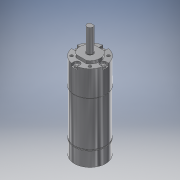
# Autodesk Inventor part: 730RPM Motor Mockup
Saved by Autodesk Inventor 2017 (Build 210142000, 142)
## iProperties
Created: 2019-01-30
Part Number: 730RPM Motor Mockup
Material: Generic
Document SubType Name: Modeling
Designer: cresswnd
Density: 1 g/cm^3
Appearance: Aluminum - Polished
Author: cresswnd
Autodesk Inventor part; units mm, degrees
ref_plane "YZ Plane" through (0, 0, 0) normal (1, 0, 0) x (0, 1, 0)
sketch "Sketch1" plane through (0, 0, 0) normal (0, 0, 1) x (1, 0, 0)
  circle A0 centre (0, 0) radius 11
  dimension "d0" = 22
  constraints: 1 centre point, 1 coincident
  measures "d0" diameter of A0
extrude "Extrusion1" add sketch "Sketch1" against normal blind 59.1
sketch "Sketch9" plane through (0, 0, 0) normal (0, 0, 1) x (1, 0, 0)
  line L0 (0, 6) -> (0, -6)
  line L1 (-3.6056, 6) -> (3.6056, 6)
  line L2 (3.6056, -6) -> (-3.6056, -6)
  arc A0 (-3.6056, 6) -> (-3.6056, -6) centre (0, 0) ccw
  arc A1 (3.6056, -6) -> (3.6056, 6) centre (0, 0) ccw
  dimension "d19" = 6
  dimension "d20" = 12
  constraints: 6 end point, 4 point on circle, 2 centre point, 1 coincident, 1 parallel, 1 perpendicular, 1 vertical
  measures "d19" distance of A0.centre L0.start
  measures "d20" distance of L0.start L0.end
extrude "Extrusion5" add sketch "Sketch9" along normal blind 2
sketch "Sketch10" plane through (0, 0, 2) normal (0, 0, 1) x (1, 0, 0)
  circle A0 centre (0, 0) radius 2.25
  dimension "d23" = 4.5
  constraints: 1 centre point, 1 coincident
  measures "d23" diameter of A0
extrude "Extrusion6" add sketch "Sketch10" along normal blind 0.2
sketch "Sketch11" plane through (0, 0, 2.2) normal (0, 0, 1) x (1, 0, 0)
  circle A0 centre (0, 0) radius 2
  dimension "d26" = 4
  constraints: 1 centre point, 1 coincident
  measures "d26" diameter of A0
extrude "Extrusion7" add sketch "Sketch11" along normal blind 16
sketch "Sketch12" plane through (0, 0, 18.2) normal (0, 0, 1) x (1, 0, 0)
  circle A0 centre (0, 0) radius 2
  line L0 (0, -2) -> (0, 1.5)
  line L1 (1.3229, 1.5) -> (-1.3229, 1.5)
  dimension "d29" = 3.5
  constraints: 4 end point, 3 point on circle, 1 centre point, 1 horizontal, 1 vertical
  measures "d29" distance of L0.start L0.end
extrude "Extrusion8" cut sketch "Sketch12" against normal blind 12 contours L1 A0
ref_plane "Work Plane1" through (0, 0, -18) normal (0, 0, 1) x (1, 0, 0)
sketch "Sketch13" plane through (0, 0, -18) normal (0, 0, 1) x (1, 0, 0)
  circle A0 centre (0, 0) radius 10.8
  circle A1 centre (0, 0) radius 11 projected
  dimension "d33" = 21.6
  constraints: 1 centre point, 1 coincident
  measures "d33" diameter of A0
extrude "Extrusion9" cut sketch "Sketch13" against normal up to surface (41.1 mm away)
ref_plane "Work Plane2" through (0, 0, -48.6) normal (0, 0, -1) x (-1, 0, 0)
sketch "Sketch14" plane through (0, 0, -48.6) normal (0, 0, -1) x (-1, 0, 0)
  circle A0 centre (0, 0) radius 10.6
  circle A1 centre (0, 0) radius 10.8 projected
  dimension "d37" = 21.2
  constraints: 1 centre point, 1 coincident
  measures "d37" diameter of A0
extrude "Extrusion10" cut sketch "Sketch14" along normal blind 0.5
fillet "Fillet1" radius 0.5 1 edges at (-11, 0, -18)
fillet "Fillet2" radius 0.25 1 edges at (-10.8, 0, -49.1)
fillet "Fillet3" radius 0.25 1 edges at (-10.8, 0, -48.6)
sketch "Sketch15" plane through (0, 0, 0) normal (0, 0, 1) x (1, 0, 0)
  circle A0 centre (0, 0) radius 11 projected
  circle A1 centre (0, 0) radius 9 construction
  circle A2 centre (0, 9) radius 1.25 construction
  circle A3 centre (-9, 0) radius 1.25 construction
  circle A4 centre (9, 0) radius 1.25 construction
  circle A5 centre (0, -9) radius 1.25 construction
  line L0 (0, 0) -> (12, 12) construction
  line L1 (0, 0) -> (16.9706, 0) construction
  line L2 (12, 12) -> (-9, -9) construction
  line L3 (0, 0) -> (10, -10) construction
  line L4 (0, 0) -> (14.1421, 0) construction
  line L5 (10, -10) -> (-10.25, 10.25) construction
  circle A6 centre (6.364, 6.364) radius 1
  circle A7 centre (-6.364, 6.364) radius 1
  circle A8 centre (-6.364, -6.364) radius 1
  circle A9 centre (6.364, -6.364) radius 1
  dimension "d43" = 18
  dimension "d44" = 2.5
  dimension "d45" = 2.5
  dimension "d46" = 2.5
  dimension "d47" = 2.5
  dimension "d48" = 45
  dimension "d49" = 45
  dimension "d50" = 2
  dimension "d51" = 2
  dimension "d52" = 2
  dimension "d53" = 2
  constraints: 12 end point, 8 centre point, 6 point on line, 2 equal length, 2 horizontal, 1 coincident, 10 other
  measures "d44" diameter of A2
  measures "d45" diameter of A3
  measures "d46" diameter of A4
  measures "d47" diameter of A5
  measures "d48" angle of L1 L0
  measures "d49" angle of L3 L4
  measures "d50" diameter of A6
  measures "d51" diameter of A7
  measures "d52" diameter of A8
  measures "d53" diameter of A9
extrude "Extrusion11" cut sketch "Sketch15" against normal blind 4 contours A6 | A7 | A8 | A9
sketch "Sketch16" plane through (0, 0, 0) normal (0, 0, 1) x (1, 0, 0)
  circle A0 centre (0, 0) radius 9 construction
  circle A1 centre (0, 0) radius 11 projected
  line L0 (-2, 9) -> (-2, 10.8167)
  line L1 (2, 9) -> (2, 10.8167)
  arc A2 (-2, 9) -> (2, 9) centre (0, 9) ccw
  line L2 (-2, -9) -> (-2, -10.8167)
  line L3 (2, -9) -> (2, -10.8167)
  arc A3 (2, -9) -> (-2, -9) centre (0, -9) ccw
  arc A4 (-9, -2) -> (-9, 2) centre (-9, 0) ccw
  line L4 (-9, 2) -> (-10.8167, 2)
  line L5 (-9, -2) -> (-10.8167, -2)
  line L6 (0, 0) -> (0, 2)
  arc A5 (9, 2) -> (9, -2) centre (9, 0) ccw
  line L7 (9, 2) -> (10.8167, 2)
  line L8 (9, -2) -> (10.8167, -2)
  arc A6 (2, 10.8167) -> (-2, 10.8167) centre (0, 0) ccw
  arc A7 (-10.8167, 2) -> (-10.8167, -2) centre (0, 0) ccw
  arc A8 (10.8167, -2) -> (10.8167, 2) centre (0, 0) ccw
  arc A9 (-2, -10.8167) -> (2, -10.8167) centre (0, 0) ccw
  dimension "d56" = 18
  dimension "d58" = 4
  constraints: 20 point on circle, 18 end point, 8 centre point, 5 symmetric about line, 3 vertical, 2 tangent, 1 coincident, 1 concentric, 1 horizontal, 1 horizontal alignment, 1 parallel, 3 other
  measures "d58" diameter of A4
extrude "Extrusion12" cut sketch "Sketch16" against normal blind 2 contours A1 L8 A5 L7 | L1 A2 L0 A1 | A1 L2 A3 L3 | L4 A4 L5 A1
sketch "Sketch17" plane through (0, 0, -2) normal (0, 0, 1) x (1, 0, 0)
  circle A0 centre (0, 0) radius 9 construction
  circle A1 centre (0, 9) radius 1.5 construction
  circle A2 centre (0, 9) radius 1.5
  circle A3 centre (-9, 0) radius 1.5
  circle A4 centre (0, -9) radius 1.5
  circle A5 centre (9, 0) radius 1.5
  dimension "d61" = 18
  dimension "d62" = 3
  dimension "d63" = 3
  dimension "d64" = 3
  dimension "d65" = 3
  constraints: 6 centre point, 4 point on circle, 2 coincident, 1 concentric
  measures "d61" diameter of A0
  measures "d62" diameter of A1
  measures "d63" diameter of A3
  measures "d64" diameter of A4
  measures "d65" diameter of A5
extrude "Extrusion13" add sketch "Sketch17" along normal blind 1.25
fillet "Fillet4" radius 0.5 4 edges at (-1.5, 9, -0.75) (7.5, 0, -0.75) (-1.5, -9, -0.75) (-10.5, 0, -0.75)
body "Solid1"
